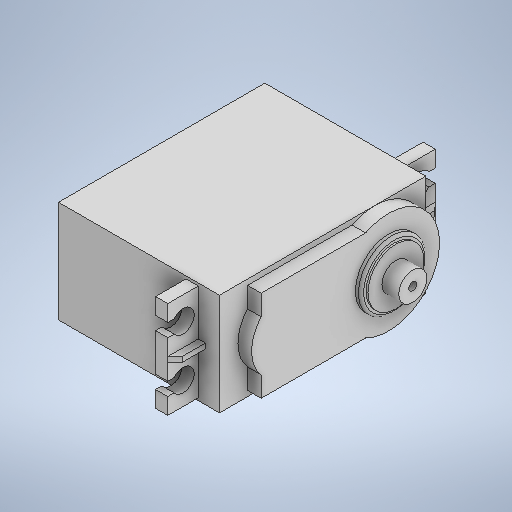
# Autodesk Inventor part: MMAE 232 Assignment 2_Servo - Dylan Tamras
Saved by Autodesk Inventor 2025.2 (Build 292293000, 293)
## iProperties
Created: 2025-01-31
Part Number: MMAE 232 Assignment 2_Servo - Dylan Tamras
Material: Generic
Document SubType Name: Modeling
Designer: Dylan
Density: 1 g/cm^3
Appearance: Default
Author: Dylan
Autodesk Inventor part; units mm, degrees
sketch "Sketch1" plane through (0, 0, 0) normal (0, 1, 0) x (-1, 0, 0)
  line L0 (0, 0) -> (31.6, 0)
  line L1 (31.6, 0) -> (31.6, 40.5)
  line L2 (31.6, 40.5) -> (0, 40.5)
  line L3 (0, 40.5) -> (0, 0)
  dimension "d0" = 31.6
  dimension "d1" = 40.5
  constraints: 8 end point, 3 perpendicular, 1 horizontal
  measures "d0" distance of L0.start L0.end
  measures "d1" distance of L0.end L1.end
extrude "Extrusion1" add sketch "Sketch1" along normal blind 20
sketch "Sketch2" plane through (0, 20, 0) normal (0, 1, 0) x (1, 0, 0)
  line L0 (-31.6, 0) -> (-31.6, -40.5) projected
  line L1 (-31.6, -13.7147) -> (-28.9372, -13.7147)
  line L2 (-28.9372, -13.7147) -> (-28.9372, -25.2066)
  line L3 (-28.9372, -25.2066) -> (-31.6, -25.2066)
  line L4 (-31.6, -25.2066) -> (-31.6, -13.7147)
  point P0 (0, 0)
  constraints: 8 end point, 2 parallel, 1 horizontal, 1 perpendicular, 1 point on line
extrude "Extrusion2" add sketch "Sketch2" along normal blind 20
sketch "Sketch3" plane through (-31.6, 0, 0) normal (-1, 0, 0) x (0, 0, 1)
  line L0 (0, 20) -> (13.7147, 20) projected
  line L1 (25.2066, 20) -> (40.5, 20) projected
  line L2 (0, 20) -> (40.5, 20)
  line L3 (40.5, 20) -> (40.5, 0)
  line L4 (40.5, 0) -> (0, 0)
  line L5 (0, 0) -> (0, 20) projected
  line L6 (0, 0) -> (0, 20)
  constraints: 8 end point, 2 collinear, 2 perpendicular
extrude "Extrusion3" add sketch "Sketch3" along normal blind 2
chamfer "Chamfer1" distance 2 angle 45 2 edges at (-33.6, 20, 20.25) (-33.6, 0, 20.25)
sketch "Sketch4" plane through (0, 40, 0) normal (0, 1, 0) x (1, 0, 0)
  line L0 (-28.9372, -13.7147) -> (-31.6, -13.7147) projected
  line L1 (-31.6, -13.7147) -> (-31.6, -25.2066) projected
  line L2 (-31.6, -25.2066) -> (-28.9372, -25.2066) projected
  line L3 (-28.9372, -25.2066) -> (-28.9372, -13.7147) projected
  point P0 (0, 0)
extrude "Extrusion4" cut sketch "Sketch4" against normal blind 20
sketch "Sketch5" plane through (0, 0, 0) normal (0, 0, -1) x (-1, 0, 0)
  line L0 (0, 0) -> (31.6, 0) projected
  line L1 (29.6, 6.65) -> (29.6, 13.35)
  line L2 (29.6, 13.35) -> (33.6, 13.35)
  line L3 (33.6, 18) -> (33.6, 2) projected
  line L4 (29.6, 6.65) -> (33.6, 6.65)
  line L5 (33.6, 6.65) -> (33.6, 13.35)
  constraints: 8 end point, 2 point on line, 1 collinear, 1 horizontal, 1 perpendicular
extrude "Extrusion5" add sketch "Sketch5" along normal blind 1.6
sketch "Sketch6" plane through (0, 0, -1.6) normal (0, 0, -1) x (-1, 0, 0)
  line L0 (33.6, 6.65) -> (29.6, 6.65) projected
  line L1 (29.6, 13.35) -> (33.6, 13.35) projected
  line L2 (33.6, 7.35) -> (33.6, 12.65)
  line L3 (33.6, 2) -> (33.6, 18) projected
  line L4 (31.6, 20) -> (33.6, 18) projected
  line L5 (33.6, 7.35) -> (29.6, 7.35)
  line L6 (33.6, 12.65) -> (29.6, 12.65)
  line L7 (29.6, 7.35) -> (29.6, 12.65)
  line L8 (29.6, 6.65) -> (29.6, 13.35) projected
  line L9 (33.1, 12.65) -> (33.1, 7.35)
  line L10 (31.6, 12.65) -> (30.6, 12.65)
  line L11 (30.6, 12.65) -> (30.6, 7.35)
  point P0 (0, 0)
  constraints: 14 end point, 4 point on line, 2 collinear, 1 horizontal, 1 midpoint, 1 perpendicular
extrude "Extrusion6" add sketch "Sketch6" along normal blind 4 contours L5 L11 L6 L9
ref_plane "Work Plane1" through (-33.1, 10, -1.6) normal (0, 1, 0) x (1, 0, 0)
sketch "Sketch7" plane through (-33.1, 10, -1.6) normal (0, 1, 0) x (1, 0, 0)
  line L0 (-0.5, 0) -> (3.5, 0) projected
  line L1 (2.5, 4) -> (0, 4) projected
  line L2 (-0.5, 0) -> (0, 4)
  line L3 (0, 0) -> (0, 4) projected
  line L4 (0, 4) -> (0, 0)
  line L5 (0, 0) -> (-0.5, 0)
  point P0 (33.1, -1.6)
  constraints: 6 end point, 1 collinear, 1 perpendicular
extrude "Extrusion7" add sketch "Sketch7" along normal blind 2.65
sketch "Sketch8" plane through (-33.1, 10, -1.6) normal (0, 1, 0) x (1, 0, 0)
  line L0 (2.5, 0) -> (2.5, 4) projected
  line L1 (3.5, -1.6) -> (3.5, 0) projected
  line L2 (2.5, 4) -> (3.5, 0)
  line L3 (3.5, 0) -> (2.5, 0)
  line L4 (2.5, 0) -> (2.5, 4)
  point P0 (33.1, -1.6)
  constraints: 6 end point, 2 perpendicular
extrude "Extrusion8" add sketch "Sketch8" along normal blind 2.65
sketch "Sketch9" plane through (-33.1, 10, -1.6) normal (0, -1, 0) x (1, 0, 0)
  line L0 (3.5, 0) -> (2.5, -4) projected
  line L1 (2.5, 0) -> (3.5, 0) projected
  line L2 (2.5, -4) -> (2.5, 0) projected
  point P0 (33.1, 1.6)
extrude "Extrusion9" add sketch "Sketch9" along normal blind 2.65
sketch "Sketch10" plane through (-33.1, 10, -1.6) normal (0, -1, 0) x (1, 0, 0)
  line L0 (-0.5, 0) -> (0, 0) projected
  line L1 (0, -4) -> (-0.5, 0) projected
  line L2 (0, 0) -> (0, -4) projected
  point P0 (33.1, 1.6)
extrude "Extrusion10" add sketch "Sketch10" along normal blind 2.65
sketch "Sketch11" plane through (0, 0, 0) normal (0, 0, -1) x (-1, 0, 0)
  line L0 (33.6, 2) -> (31.6, 0) projected
  line L1 (6.55, 0.5) -> (6.55, 19.5)
  line L2 (6.55, 0.5) -> (2.75, 0.5)
  line L3 (2.75, 0.5) -> (2.75, 19.5)
  line L4 (2.75, 19.5) -> (6.55, 19.5)
  point P0 (31.6, 20)
  dimension "d37" = 3.8
  constraints: 8 end point, 2 perpendicular, 1 horizontal, 1 vertical
  measures "d37" distance of L1.start L2.end
extrude "Extrusion11" add sketch "Sketch11" along normal blind 6
sketch "Sketch12" plane through (-2.75, 0.5, 0) normal (1, 0, 0) x (0, 0, -1)
  line L0 (0, 19) -> (0, 0) projected
  line L1 (0, 19) -> (6, 19) projected
  line L2 (0, 19) -> (6, 19)
  circle A0 centre (3, 14.5) radius 2.18
  line L3 (6, 15.8) -> (4.75, 15.8)
  line L4 (6, 13.2) -> (4.75, 13.2)
  line L5 (6, 13.2) -> (6, 15.8)
  circle A1 centre (3, 4.5) radius 2.18
  line L6 (6, 5.8) -> (4.75, 5.8)
  line L7 (6, 3.2) -> (4.75, 3.2)
  line L8 (6, 3.2) -> (6, 5.8)
  point P0 (0, -0.5)
  dimension "d40" = 3.2
  dimension "d43" = 4.36
  dimension "d45" = 7.4
  dimension "d47" = 4.36
  constraints: 14 end point, 4 point on circle, 3 horizontal, 2 centre point, 1 perpendicular
  measures "d40" distance of L1.end L3.start
  measures "d43" diameter of A0
  measures "d45" distance of L4.start L6.start
  measures "d47" diameter of A1
extrude "Extrusion12" cut sketch "Sketch12" against normal blind 6
sketch "Sketch13" plane through (-2.75, 0.5, 0) normal (1, 0, 0) x (0, 0, -1)
  line L0 (6, 13.2) -> (4.75, 13.2) projected
  arc A0 (4.75, 15.8) -> (4.75, 13.2) centre (3, 14.5) ccw projected
  line L1 (4.75, 15.8) -> (6, 15.8) projected
  line L2 (6, 19) -> (6, 15.8) projected
  line L3 (0, 19) -> (6, 19) projected
  line L4 (0, 0) -> (0, 19) projected
  line L5 (0, 0) -> (6, 0) projected
  line L6 (6, 3.2) -> (6, 0) projected
  line L7 (6, 3.2) -> (4.75, 3.2) projected
  arc A1 (4.75, 5.8) -> (4.75, 3.2) centre (3, 4.5) ccw projected
  line L8 (4.75, 5.8) -> (6, 5.8) projected
  line L9 (6, 13.2) -> (6, 5.8) projected
  point P0 (0, -0.5)
extrude "Extrusion13" cut sketch "Sketch13" against normal blind 1.4
sketch "Sketch14" plane through (-4.15, 0.5, 0) normal (1, 0, 0) x (0, 0, -1)
  line L0 (0, 19) -> (6, 19) projected
  line L1 (6, 19) -> (6, 15.8) projected
  line L2 (6, 13.2) -> (6, 5.8) projected
  line L3 (0, 9) -> (0, 10)
  line L4 (0, 10) -> (4.5, 10)
  line L5 (4.5, 10) -> (4.5, 9)
  line L6 (0, 9) -> (4.5, 9)
  point P0 (0, -0.5)
  dimension "d55" = 4.5
  constraints: 8 end point
  measures "d55" distance of L3.end L4.end
extrude "Extrusion14" add sketch "Sketch14" along normal blind 1.4
ref_plane "Work Plane2" through (-4.15, 10, -4.5) normal (0, -1, 0) x (1, 0, 0)
sketch "Sketch15" plane through (-4.15, 10, -4.5) normal (0, -1, 0) x (1, 0, 0)
  line L0 (0, -1.5) -> (0, -0.25) projected
  line L1 (1.4, 0) -> (0, -1.5)
  line L2 (0, -1.5) -> (0, 0)
  line L3 (0, 0) -> (1.4, 0)
  point P0 (4.15, 4.5)
  constraints: 6 end point, 1 collinear, 1 perpendicular
extrude "Extrusion15" add sketch "Sketch15" along normal blind 0.5
sketch "Sketch16" plane through (-4.15, 10, -4.5) normal (0, 1, 0) x (1, 0, 0)
  line L0 (1.4, 0) -> (0, 0) projected
  line L1 (0, 1.5) -> (1.4, 0) projected
  line L2 (0, 0) -> (0, 1.5) projected
  point P0 (4.15, -4.5)
extrude "Extrusion16" add sketch "Sketch16" along normal blind 0.5
ref_plane "Work Plane3" through (0, 0, 20.25) normal (0, 0, -1) x (-1, 0, 0)
mirror "Mirror1" about plane through (0, 0, 20.25) normal (0, 0, -1) of "Extrusion12", "Extrusion13", "Extrusion14", "Extrusion15", "Extrusion11"
sketch "Sketch17" plane through (-4.15, 10, 45) normal (0, 1, 0) x (1, 0, 0)
  line L0 (1.4, 0) -> (0, 0) projected
  line L1 (0, -1.5) -> (0, 0) projected
  line L2 (0, -1.5) -> (1.4, 0) projected
  point P0 (4.15, 45)
extrude "Extrusion17" add sketch "Sketch17" along normal blind 0.5
sketch "Sketch18" plane through (0, 0, 40.5) normal (1, 0, 0) x (0, 0, -1)
  circle A0 centre (30.5, 10) radius 10
  line L0 (26, 1.07) -> (5.5, 1.07)
  line L1 (26, 18.93) -> (5.5, 18.93)
  circle A1 centre (11.02, 10) radius 7.4
  line L2 (5.5, 1.07) -> (5.5, 5.0716)
  line L3 (5.5, 18.93) -> (5.5, 14.9284)
  point P0 (40.5, 20)
  point P1 (25.9994, 18.93)
  point P2 (25.9994, 1.07)
  dimension "d68" = 20
  dimension "d71" = 14.8
  constraints: 8 end point, 2 centre point, 2 point on circle, 1 point on line, 1 vertical
  measures "d68" diameter of A0
  measures "d71" diameter of A1
extrude "Extrusion18" add sketch "Sketch18" along normal blind 2.68
sketch "Sketch19" plane through (2.68, 0, 40.5) normal (1, 0, 0) x (0, 0, -1)
  line L0 (40.5, 6.65) -> (40.5, 13.35) projected
  circle A0 centre (30.5, 10) radius 6.5
  point P0 (40.5, 0)
  dimension "d75" = 13
  constraints: 1 centre point
  measures "d75" diameter of A0
extrude "Extrusion19" add sketch "Sketch19" along normal blind 1.1
sketch "Sketch20" plane through (3.78, 10, 10) normal (1, 0, 0) x (0, 0, -1)
  circle A0 centre (0, 0) radius 5.5
  point P0 (10, -10)
  dimension "d79" = 11
  constraints: 1 centre point
  measures "d79" diameter of A0
extrude "Extrusion20" add sketch "Sketch20" along normal blind 0.35
sketch "Sketch21" plane through (4.13, 10, 10) normal (1, 0, 0) x (0, 0, -1)
  circle A0 centre (0, 0) radius 2.75
  point P0 (10, -10)
  dimension "d82" = 5.5
  constraints: 1 centre point
  measures "d82" diameter of A0
extrude "Extrusion21" add sketch "Sketch21" along normal blind 3.3
fillet "Fillet1" radius 0.5 1 edges at (3.78, 10, 16.5)
sketch "Sketch22" plane through (7.43, 10, 10) normal (1, 0, 0) x (0, 0, -1)
  circle A0 centre (0, 0) radius 1
  dimension "d86" = 2
  constraints: 1 centre point
  measures "d86" diameter of A0
hole "Hole1" at (7.43, 10, 10) direction (-1, 0, 0) diameter 1.567 depth 6 tip angle 118 thread size "M2x0.4" class "6H" standard "ANSI Metric M Profile"
sketch "Sketch23" plane through (0, 0, 40.5) normal (0, 0, 1) x (1, 0, 0)
  line L0 (-33.6, 18) -> (-31.6, 20) projected
  line L1 (-33.6, 18) -> (-29.6, 18) construction
  line L2 (0, 20) -> (-31.6, 20) projected
  line L3 (-31.6, 20) -> (-32.5985, 20)
  line L4 (-33.6, 2) -> (-33.6, 18) projected
  line L5 (-33.6, 18) -> (-32.5985, 20)
  line L6 (-33.6, 2) -> (-29.6, 2) construction
  line L7 (-31.6, 0) -> (-32.5985, 0)
  line L8 (-31.6, 0) -> (-33.6, 2) projected
  line L9 (-33.6, 2) -> (-32.5985, 0)
  point P0 (0, 0)
  constraints: 12 end point, 4 horizontal
extrude "Extrusion22" add sketch "Sketch23" against normal blind 40.5
sketch "Sketch24" plane through (0, 0, 40.5) normal (0, 0, 1) x (1, 0, 0)
  line L0 (-33.6, 18) -> (-32.5985, 20) projected
  line L1 (-32.5985, 20) -> (-33.6, 20)
  line L2 (-33.6, 20) -> (-33.6, 18)
  line L3 (-32.5985, 0) -> (-33.6, 2) projected
  line L4 (-33.6, 2) -> (-33.6, 0)
  line L5 (-33.6, 0) -> (-32.5985, 0)
  point P0 (0, 0)
  constraints: 8 end point, 2 perpendicular, 1 horizontal, 1 vertical
extrude "Extrusion23" add sketch "Sketch24" against normal blind 40.5
chamfer "Chamfer2" distance 2 angle 45 2 edges at (-33.6, 20, 20.25) (-33.6, 0, 20.25)
chamfer "Chamfer3" distance 2 angle 63.4 1 edges at (-33.6, 10, 40.5) measured on face at (-23.25, 6.8333, 40.5)
body "Solid1"
